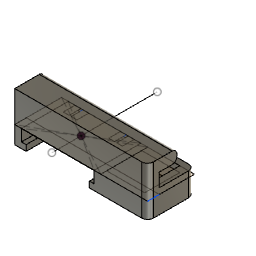
drill battery holder (Autodesk Fusion 360 design; units mm, degrees)
Autodesk Fusion 360 part; units mm, degrees
sketch "Sketch1" plane through (0, 0, 0) normal (0, 0, 1) x (1, 0, 0)
  line L0 (31, 20) -> (-31, 20)
  line L1 (-31, 20) -> (-31, -20)
  line L2 (-31, -20) -> (31, -20)
  line L3 (31, -20) -> (31, 20)
  line L4 (31, 20) -> (-31, -20) construction
  line L5 (-31, 20) -> (31, -20) construction
  line L6 (36.75, 20) -> (-36.75, 20)
  line L7 (-36.75, 20) -> (-36.75, -20)
  line L8 (-36.75, -20) -> (36.75, -20)
  line L9 (36.75, -20) -> (36.75, 20)
  line L10 (36.75, 20) -> (-36.75, -20) construction
  line L11 (-36.75, 20) -> (36.75, -20) construction
  line L12 (36.75, -20) -> (76.75, -20)
  line L13 (76.75, -20) -> (76.75, 20)
  line L14 (76.75, 20) -> (36.75, 20)
  line L15 (36.75, 20) -> (36.75, -20)
  line L16 (36.75, -15) -> (69.25, -15)
  line L17 (69.25, -15) -> (69.25, 15)
  line L18 (69.25, 15) -> (36.75, 15)
  line L19 (36.75, 15) -> (36.75, -15)
  line L20 (-36.75, -20) -> (76.75, -20)
  line L21 (76.75, -20) -> (76.75, -10)
  line L22 (76.75, -10) -> (-36.75, -10)
  line L23 (-36.75, -10) -> (-36.75, -20)
  line L24 (-20.25, 20) -> (-25.25, 20)
  line L25 (-25.25, 20) -> (-25.25, 10)
  line L26 (-25.25, 10) -> (-20.25, 10)
  line L27 (-20.25, 10) -> (-20.25, 20)
  line L28 (-18.55, 20) -> (-13.55, 20)
  line L29 (-13.55, 20) -> (-13.55, 10)
  line L30 (-13.55, 10) -> (-18.55, 10)
  line L31 (-18.55, 10) -> (-18.55, 20)
  line L32 (-20.25, 20) -> (-18.55, 20)
  line L33 (-18.55, 20) -> (-18.55, 17.5)
  line L34 (-18.55, 17.5) -> (-20.25, 17.5)
  line L35 (-20.25, 17.5) -> (-20.25, 20)
  line L36 (0, -25) -> (0, 65)
  line L37 (25.25, 10) -> (20.25, 10)
  line L38 (20.25, 20) -> (18.55, 20)
  line L39 (13.55, 10) -> (18.55, 10)
  line L40 (20.25, 10) -> (20.25, 20)
  line L41 (18.55, 20) -> (13.55, 20)
  line L42 (18.55, 20) -> (18.55, 17.5)
  line L43 (18.55, 10) -> (18.55, 20)
  line L44 (20.25, 20) -> (25.25, 20)
  line L45 (25.25, 20) -> (25.25, 10)
  line L46 (18.55, 17.5) -> (20.25, 17.5)
  line L47 (20.25, 17.5) -> (20.25, 20)
  line L48 (13.55, 20) -> (13.55, 10)
  dimension "d1" = 62
  dimension "d2" = 40
  dimension "d3" = 73.5
  dimension "d12" = 40
  dimension "d13" = 40
  dimension "d14" = 5
  dimension "d15" = 5
  dimension "d16" = 7.5
  dimension "d23" = 10
  dimension "d35" = 5
  dimension "d36" = 10
  dimension "d37" = 5
  dimension "d38" = 10
  dimension "d39" = 2.5
  dimension "d42" = 40.5
  dimension "d43" = 37.1
  constraint perpendicular L0 L1
  constraint parallel L0 L2
  constraint parallel L1 L3
  constraint horizontal L0
  constraint coincident L4 origin
  constraint coincident L5 origin
  constraint perpendicular L6 L7
  constraint parallel L6 L8
  constraint parallel L7 L9
  constraint horizontal L6
  constraint coincident L10 origin
  constraint coincident L11 origin
  constraint horizontal L12
  constraint vertical L13
  constraint horizontal L14
  constraint vertical L15
  constraint horizontal L16
  constraint vertical L17
  constraint horizontal L18
  constraint vertical L19
  constraint coincident L9 L16.start
  constraint horizontal L20
  constraint vertical L21
  constraint horizontal L22
  constraint vertical L23
  constraint horizontal L24
  constraint vertical L25
  constraint horizontal L26
  constraint vertical L27
  constraint coincident L0 L24.start
  constraint coincident L6 L24.start
  constraint horizontal L28
  constraint vertical L29
  constraint horizontal L30
  constraint vertical L31
  constraint coincident L6 L28.start
  constraint horizontal L32
  constraint vertical L33
  constraint horizontal L34
  constraint vertical L35
  constraint perpendicular L2 L36
  constraint midpoint L0 L36
  constraint symmetric L24.start L36 L38.start
  constraint symmetric L24.end L36 L44.end
  constraint symmetric L25.end L36 L37.start
  constraint symmetric L26.end L36 L37.end
  constraint symmetric L28.start L36 L38.end
  constraint symmetric L28.end L36 L41.end
  constraint symmetric L29.end L36 L39.start
  constraint symmetric L30.end L36 L39.end
  constraint symmetric L33.end L36 L42.end
  constraint symmetric L34.end L36 L46.end
  measures "d1" distance of L1.end L2.end
  measures "d2" distance of L0.end L1.end
  measures "d3" distance of L7.end L8.end
  measures "d12" distance of L8.end L12.end
  measures "d13" distance of L8.end L6.start
  measures "d14" distance of L12 L16
  measures "d15" distance of L14 L18
  measures "d16" distance of L13 L17
  measures "d23" distance of L7.end L22.end
  measures "d35" distance of L24.start L24.end
  measures "d36" distance of L24.start L26.end
  measures "d37" distance of L28.start L28.end
  measures "d38" distance of L28 L30
  measures "d39" distance of L24.start L34.end
  measures "d42" distance of L27 L40
  measures "d43" distance of L31 L43
extrude "Extrude6" add sketch "Sketch1" along normal blind 16.6 contours L3 L8 L9 L15 L19 L20 L22 | L2 L3 L8 L20 L22 L36 | L9 L15 L16 L17 L19 L22 | L1 L2 L8 L20 L22 L36 | L9 L12 L13 L15 L16 L17 L20 L21 L22 | L1 L7 L8 L20 L22 L23 makes body 1
extrude "Extrude2" add sketch "Sketch1" against normal blind 15 separate body contours L3 L6 L9 L15 L19 L22 | L3 L8 L9 L15 L19 L20 L22 | L1 L6 L7 L22 | L1 L7 L8 L20 L22 L23 makes body 2 at (31, -6.6667, -10) makes body 3 at (-31, 6.6667, -10)
extrude "Extrude1" add sketch "Sketch1" along normal blind 5 separate body contours L0 L3 L6 L22 L36 L37 L39 L40 L43 L45 L46 L48 | L3 L6 L9 L15 L19 L22 | L0 L6 L37 L40 L44 L45 L47 | L3 L8 L9 L15 L19 L20 L22 | L2 L3 L8 L20 L22 L36 | L0 L6 L38 L40 L42 L43 L46 L47 | L1 L2 L8 L20 L22 L36 | L0 L1 L6 L22 L25 L26 L27 L29 L30 L31 L34 L36 | L0 L6 L39 L41 L42 L43 L48 | L1 L6 L7 L22 | L1 L7 L8 L20 L22 L23 | L0 L6 L28 L29 L30 L31 L33 | L0 L6 L24 L25 L26 L27 L35 | L0 L6 L27 L31 L32 L33 L34 L35 makes body 4
sketch "Sketch2" plane through (0, -20, 0) normal (0, -1, 0) x (1, 0, 0)
  line L0 (36.75, 0) -> (31, 0)
  line L1 (31, 0) -> (31, -15)
  line L2 (31, -15) -> (36.75, -15)
  line L3 (36.75, -15) -> (36.75, 0)
  line L4 (31, -15) -> (27, -15)
  line L5 (27, -15) -> (27, -10)
  line L6 (27, -10) -> (31, -10)
  line L7 (31, -10) -> (31, -15)
  line L8 (0, 30) -> (0, -50)
  line L9 (-31, -15) -> (-27, -15)
  line L10 (-31, -15) -> (-36.75, -15)
  line L11 (-31, -10) -> (-31, -15)
  line L12 (-27, -10) -> (-31, -10)
  line L13 (-27, -15) -> (-27, -10)
  dimension "d8" = 4
  dimension "d9" = 5
  constraint horizontal L4
  constraint vertical L5
  constraint horizontal L6
  constraint vertical L7
  constraint coincident L1.end L2.start
  constraint vertical L8
  constraint symmetric L1.end L8 L9.start
  constraint symmetric L2.end L8 L10.end
  constraint symmetric L4.end L8 L9.end
  constraint symmetric L5.end L8 L12.start
  constraint symmetric L6.end L8 L11.start
  measures "d8" distance of L1.end L4.end
  measures "d9" distance of L1.end L6.end
extrude "Extrude3" add sketch "Sketch2" against normal up to surface (40 mm away) contours L1 L4 L5 L6 L7 | L9 L11 L12 L13 bodies 2 3 4
extrude "Extrude4" add sketch "Sketch1" along normal up to surface (-15 mm away) and the other way up to surface (-5 mm away) contours L9 L13 L14 L15 L17 L18 L22 | L9 L12 L13 L15 L16 L17 L20 L21 L22 bodies 2 4
sketch "Sketch3" plane through (0, 0, -15) normal (0, 0, -1) x (1, 0, 0)
  line L0 (76.75, 20) -> (27, 20)
  line L1 (27, 20) -> (27, -20)
  line L2 (27, -20) -> (76.75, -20)
  line L3 (76.75, -20) -> (76.75, 20)
  line L4 (36.75, 15) -> (69.25, 15)
  line L5 (69.25, 15) -> (69.25, -15)
  line L6 (69.25, -15) -> (36.75, -15)
  line L7 (36.75, -15) -> (36.75, 15)
extrude "Extrude5" add sketch "Sketch3" against normal blind 5 contours L4 L5 L6 L7 bodies 2
sketch "Sketch4" plane through (0, 0, 16.6) normal (0, 0, 1) x (-1, 0, 0)
  line L0 (36.75, 10) -> (36.75, 20)
  line L1 (36.75, 20) -> (-76.75, 20)
  line L2 (-76.75, 20) -> (-76.75, 10)
  line L3 (-76.75, 10) -> (36.75, 10)
  line L4 (36.75, 20) -> (-76.75, 20)
  line L5 (-76.75, 20) -> (-76.75, -5)
  line L6 (-76.75, -5) -> (36.75, -5)
  line L7 (36.75, -5) -> (36.75, 20)
  line L8 (36.75, 10) -> (36.75, 20)
  line L9 (36.75, 20) -> (-76.75, 20)
  line L10 (-76.75, 20) -> (-76.75, 10)
  line L11 (-76.75, 10) -> (36.75, 10)
  dimension "d26" = 25
  constraint horizontal L4
  constraint vertical L5
  constraint horizontal L6
  constraint vertical L7
  constraint coincident L0.end L1.start
  measures "d26" distance of L0.end L6.end
extrude "Extrude7" add sketch "Sketch4" along normal blind 10 bodies 1
fillet "Fillet1" radius 4 2 edges at (20, 5, 16.6) (20, 5, 26.6) on bodies 1
fillet "Fillet2" radius 5 3 edges at (76.75, 20, -5) (76.75, -20, -5) (76.75, -20, 13.3) on bodies 1 2
combine "Combine1" operation add target body 1 tool bodies 2 3
extrude "Extrude8" add sketch "Sketch1" against normal blind 6.3 contours L0 L6 L37 L40 L44 L45 L47 | L0 L6 L38 L40 L42 L43 L46 L47 | L0 L6 L39 L41 L42 L43 L48 | L0 L6 L28 L29 L30 L31 L33 | L0 L6 L24 L25 L26 L27 L35 | L0 L6 L27 L31 L32 L33 L34 L35 bodies 1
